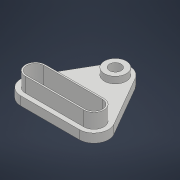
# Autodesk Inventor part: Offset
Saved by Autodesk Inventor 2022.4 (Build 264492000, 492)
## iProperties
Created: 2016-01-25
Part Number: Offset
Material: Generic
Document SubType Name: Modeling
Designer: jmacmillan
Density: 1 g/cm^3
Appearance: Default
Mass: 11.8242 g
Surface Area: 81.59 cm^2
Volume: 11.8242 cm^3
Author: jmacmillan
Autodesk Inventor part; units mm, degrees
ref_plane "YZ Plane" through (0, 0, 0) normal (1, 0, 0) x (0, 1, 0)
ref_plane "XZ Plane" through (0, 0, 0) normal (0, 1, 0) x (-1, 0, 0)
ref_plane "XY Plane" through (0, 0, 0) normal (0, 0, 1) x (1, 0, 0)
sketch "Sketch1" plane through (0, 0, 0) normal (0, 0, 1) x (1, 0, 0)
  arc A0 (8.6603, 39.641) -> (-8.6603, 39.641) centre (0, 34.641) ccw
  arc A1 (-28.6603, 5) -> (-20, -10) centre (-20, 0) ccw
  arc A2 (20, -10) -> (28.6603, 5) centre (20, 0) ccw
  line L0 (-8.6603, 39.641) -> (-28.6603, 5)
  line L1 (-20, -10) -> (20, -10)
  line L2 (28.6603, 5) -> (8.6603, 39.641)
  circle A3 centre (0, 34.641) radius 7.5
  line L3 (0, 56.0692) -> (0, -23.9282) projected
  line L4 (-46.1865, 0) -> (46.1865, 0) projected
  circle A4 centre (0, 34.641) radius 4
  point P0 (0, 0)
  dimension "d0" = 10
  dimension "d1" = 40
  dimension "d2" = 15
  dimension "d7" = 8
  constraints: 8 point on circle, 6 end point, 6 tangent, 5 centre point, 5 point on line, 2 coincident, 2 equal length, 2 equal radius
  measures "d0" radius of A2
  measures "d1" distance of L0.start L0.end
  measures "d2" diameter of A3
  measures "d7" diameter of A4
extrude "Extrusion1" add sketch "Sketch1" along normal mid plane 6
extrude "Extrusion2" add sketch "Sketch1" along normal mid plane 15 contours L3 A4 A3 | A3 L3 A4 | A4 L3 | L3 A4
extrude "Extrusion3" cut sketch "Sketch1" along normal through all both and the other way through all contours A4 L3 | L3 A4
sketch "Sketch2" plane through (0, 0, 3) normal (0, 0, 1) x (1, 0, 0)
  circle A0 centre (0, 34.641) radius 7.5 projected
  line L0 (-8.6603, 39.641) -> (-28.6603, 5) projected
  arc A1 (-28.6603, 5) -> (-20, -10) centre (-20, 0) ccw projected
  line L1 (-20, -10) -> (20, -10) projected
  arc A2 (20, -10) -> (28.6603, 5) centre (20, 0) ccw projected
  line L2 (28.6603, 5) -> (8.6603, 39.641) projected
  arc A3 (-20, 6.85) -> (-20, -6.85) centre (-20, 0) ccw
  line L3 (-20, -6.85) -> (20, -6.85)
  arc A4 (20, -6.85) -> (20, 6.85) centre (20, 0) ccw
  line L4 (-20, 6.85) -> (20, 6.85)
  arc A5 (8.6603, 39.641) -> (-8.6603, 39.641) centre (0, 34.641) ccw projected
  point P0 (0, 0)
  dimension "d10" = 3.15
  constraints: 4 end point, 4 point on circle, 2 centre point, 1 horizontal, 1 tangent, 2 other
  measures "d10" distance between parallel lines of L1 L3
extrude "Extrusion4" add sketch "Sketch2" along normal blind 10 contours L4 A4 L3 A3
sketch "Sketch3" plane through (0, 0, 13) normal (0, 0, 1) x (1, 0, 0)
  line L0 (-20, -6.85) -> (20, -6.85) projected
  arc A0 (20, -6.85) -> (20, 6.85) centre (20, 0) ccw projected
  line L1 (20, 6.85) -> (-20, 6.85) projected
  arc A1 (-20, 6.85) -> (-20, -6.85) centre (-20, 0) ccw projected
  line L2 (20, -5.85) -> (-20, -5.85)
  arc A2 (-20, 5.85) -> (-20, -5.85) centre (-20, 0) ccw
  line L3 (-20, 5.85) -> (20, 5.85)
  arc A3 (20, -5.85) -> (20, 5.85) centre (20, 0) ccw
  point P0 (0, 0)
  dimension "d13" = 1
  constraints: 4 end point, 4 point on circle, 2 centre point, 3 other
  measures "d13" distance between parallel lines of L0 L2
extrude "Extrusion5" cut sketch "Sketch3" against normal through all contours L2 A2 L3 A3
body "Solid1"
